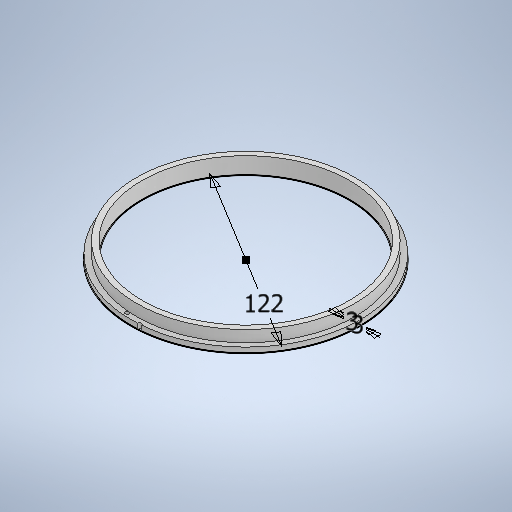
# Autodesk Inventor part: 122mm-CoilForm
Saved by Autodesk Inventor 2025.2 (Build 292293000, 293)
## iProperties
Created: 2025-05-18
Part Number: 122mm-CoilForm
Material: Generic
Document SubType Name: Modeling
Designer: user
Density: 1 g/cm^3
Appearance: Default
Author: user
## iProperties of the stored document 122mm-CoilForm_3DPrint.ipt
Created: 2025-05-18
Part Number: 122mm-CoilForm_3DPrint
Material: Generic
Document SubType Name: Modeling
Designer: user
Density: 1 g/cm^3
Appearance: Default
Author: user
Autodesk Inventor part; units mm, degrees
ref_plane "YZ Plane" through (0, 0, 0) normal (1, 0, 0) x (0, 1, 0)
ref_plane "XZ Plane" through (0, 0, 0) normal (0, 1, 0) x (-1, 0, 0)
ref_plane "XY Plane" through (0, 0, 0) normal (0, 0, 1) x (1, 0, 0)
sketch "Sketch1" plane through (0, 0, 0) normal (0, 1, 0) x (-1, 0, 0)
  circle A0 centre (0, 0) radius 61
  circle A1 centre (0, 0) radius 58
  circle A2 centre (0, 0) radius 64
  dimension "d0" = 122
  dimension "d1" = 3
  dimension "d2" = 3
  constraints: 3 centre point, 1 coincident
  measures "d0" diameter of A0
  measures "d1" radial gap between concentric circles of A0 A1
  measures "d2" radial gap between concentric circles of A0 A2
extrude "Extrusion1" add sketch "Sketch1" along normal blind 9.4 contours A0
extrude "Extrusion2" add sketch "Sketch1" along normal blind 3 contours A2
sketch "Sketch2" plane through (0, 3, 0) normal (0, 1, 0) x (1, 0, 0)
  circle A0 centre (-4.5, -61.8365) radius 1
  circle A1 centre (0, 0) radius 61 projected
  circle A2 centre (0, 0) radius 63 construction
  circle A3 centre (4.5, -63.8416) radius 1
  dimension "d7" = 2
  dimension "d8" = 4.5
  dimension "d9" = 4.5
  constraints: 3 centre point, 3 tangent, 1 coincident, 1 equal radius
  measures "d7" diameter of A0
  measures "d8" horizontal distance of A0.centre point (0, 0)
  measures "d9" horizontal distance of A3.centre point (0, 0)
extrude "Extrusion3" cut sketch "Sketch2" against normal up to surface (3 mm away) contours A0 | A3
body "Solid1"
